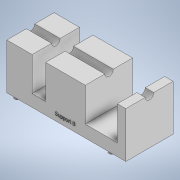
# Autodesk Inventor part: support_2
Saved by Autodesk Inventor 2021 (Build 250183000, 183)
## iProperties
Created: 2021-04-13
Part Number: support_2
Material: Generic
Document SubType Name: Modeling
Designer: Jawal
Density: 1 g/cm^3
Appearance: Default
Author: Jawal
Autodesk Inventor part; units mm, degrees
note: some values were not read from the file. Chosen so that the rebuilt part matches the saved one: direction of "Emboss1".
ref_plane "YZ Plane" through (0, 0, 0) normal (1, 0, 0) x (0, 1, 0)
ref_plane "XZ Plane" through (0, 0, 0) normal (0, 1, 0) x (-1, 0, 0)
ref_plane "XY Plane" through (0, 0, 0) normal (0, 0, 1) x (1, 0, 0)
sketch "Sketch7" plane through (0, 0, 0) normal (0, 1, 0) x (-1, 0, 0)
  line L0 (35, 14.012) -> (-35.5, 14.012)
  line L1 (-35.5, 14.012) -> (-35.5, -14.012)
  line L2 (-35.5, -14.012) -> (35, -14.012)
  line L3 (35, -14.012) -> (35, 14.012)
  point P0 (0, 0)
  dimension "d32" = 70.5
  dimension "d34" = 28.024
  dimension "d35" = 14.012
  constraints: 8 end point, 2 parallel, 1 horizontal, 1 perpendicular
  measures "d32" distance of L1.end L2.end
  measures "d34" distance of L2.end L0.start
  measures "d35" distance from line of L2 point (0, 0)
extrude "Extrusion3" add sketch "Sketch7" along normal blind 27.147
sketch "Sketch8" plane through (-35, 0, 14.012) normal (0, 0, 1) x (1, 0, 0)
  line L0 (70.5, 27.147) -> (0, 27.147) projected
  line L1 (15, 27.147) -> (23, 27.147)
  line L2 (23, 27.147) -> (23, 7.147)
  line L3 (23, 7.147) -> (15, 7.147)
  line L4 (15, 7.147) -> (15, 27.147)
  line L5 (0, 0) -> (0, 27.147) projected
  line L6 (46.5, 27.147) -> (65.5, 27.147)
  line L7 (65.5, 27.147) -> (65.5, 7.147)
  line L8 (65.5, 7.147) -> (46.5, 7.147)
  line L9 (46.5, 7.147) -> (46.5, 27.147)
  line L10 (70.5, 0) -> (70.5, 27.147) projected
  point P0 (35, 0)
  point P1 (23, 27.147)
  dimension "d39" = 20
  dimension "d40" = 15
  dimension "d41" = 8
  dimension "d42" = 46.5
  dimension "d44" = 5
  constraints: 16 end point, 4 parallel, 2 horizontal, 2 perpendicular, 2 point on line
  measures "d39" distance of L1.end L2.end
  measures "d40" distance between parallel lines of L5 L4
  measures "d41" distance of L2.end L3.end
  measures "d42" distance between parallel lines of L9 L5
  measures "d44" distance between parallel lines of L7 L10
extrude "Extrusion4" cut sketch "Sketch8" against normal through all
sketch "Sketch9" plane through (-35, 0, -14.012) normal (-1, 0, 0) x (0, 0, 1)
  line L0 (0, 27.147) -> (28.024, 27.147) projected
  arc A0 (11.512, 27.147) -> (16.512, 27.147) centre (14.012, 27.147) ccw
  point P0 (14.012, 0)
  dimension "d47" = 5
  constraints: 2 point on circle, 2 point on line, 1 centre point, 1 midpoint
  measures "d47" diameter of A0
extrude "Extrusion5" cut sketch "Sketch9" against normal through all
sketch "Sketch10" plane through (0, 0, 0) normal (0, -1, 0) x (1, 0, 0)
  circle A0 centre (-32.5, 10.512) radius 1.5
  line L0 (-35, -14.012) -> (-35, 14.012) projected
  circle A1 centre (23.5, 10.512) radius 1.5
  line L1 (35.5, 14.012) -> (35.5, -14.012) projected
  line L2 (-35, 14.012) -> (35.5, 14.012) projected
  point P0 (0, 0)
  dimension "d50" = 3
  dimension "d51" = 2.5
  dimension "d52" = 3
  dimension "d56" = 56
  dimension "d57" = 3.5
  dimension "d58" = 3.5
  constraints: 2 centre point
  measures "d50" diameter of A0
  measures "d51" distance from line of L0 A0.centre
  measures "d52" diameter of A1
  measures "d56" distance of A1.centre A0.centre
  measures "d57" distance from line of L2 A0.centre
  measures "d58" distance from line of L2 A1.centre
extrude "Extrusion6" add sketch "Sketch10" along normal blind 3
sketch "Sketch11" plane through (-35, 0, 14.012) normal (0, 0, 1) x (1, 0, 0)
  line L0 (28.6031, 5.0261) -> (50.5352, 5.0261) construction
  line L1 (50.5352, 5.0261) -> (50.5352, -0.6092) construction
  line L2 (50.5352, -0.6092) -> (28.6031, -0.6092) construction
  line L3 (28.6031, -0.6092) -> (28.6031, 5.0261) construction
  spline S0 degree 2 poles (29.3633, 2.9548) (29.1461, 2.9548) (28.8414, 3.0455) (28.7069, 3.1104) knots 0 0 0 1 2 2 2
  line L4 (28.7069, 3.1104) -> (28.7069, 3.4442)
  line L5 (28.7069, 3.4442) -> (28.7263, 3.4442)
  spline S1 degree 2 poles (28.7263, 3.4442) (28.8576, 3.3211) (29.1899, 3.1849) (29.3438, 3.1849) knots 0 0 0 1 2 2 2
  spline S2 degree 2 poles (29.3438, 3.1849) (29.5643, 3.1849) (29.7895, 3.3681) (29.7895, 3.5188) knots 0 0 0 1 2 2 2
  spline S3 degree 2 poles (29.7895, 3.5188) (29.7895, 3.6387) (29.6712, 3.7878) (29.5432, 3.8251) knots 0 0 0 1 2 2 2
  spline S4 degree 2 poles (29.5432, 3.8251) (29.4508, 3.8511) (29.2968, 3.8867) (29.1818, 3.9159) knots 0 0 0 1 2 2 2
  spline S5 degree 2 poles (29.1818, 3.9159) (29.078, 3.9434) (28.9143, 4.0261) (28.8511, 4.0925) knots 0 0 0 1 2 2 2
  spline S6 degree 2 poles (28.8511, 4.0925) (28.7895, 4.159) (28.7215, 4.3373) (28.7215, 4.454) knots 0 0 0 1 2 2 2
  spline S7 degree 2 poles (28.7215, 4.454) (28.7215, 4.6971) (29.1007, 5.0261) (29.3941, 5.0261) knots 0 0 0 1 2 2 2
  spline S8 degree 2 poles (29.3941, 5.0261) (29.5626, 5.0261) (29.8608, 4.9596) (29.9889, 4.8964) knots 0 0 0 1 2 2 2
  line L6 (29.9889, 4.8964) -> (29.9889, 4.5788)
  line L7 (29.9889, 4.5788) -> (29.9694, 4.5788)
  spline S9 degree 2 poles (29.9694, 4.5788) (29.8738, 4.6663) (29.5756, 4.796) (29.4119, 4.796) knots 0 0 0 1 2 2 2
  spline S10 degree 2 poles (29.4119, 4.796) (29.2271, 4.796) (28.9986, 4.6225) (28.9986, 4.4815) knots 0 0 0 1 2 2 2
  spline S11 degree 2 poles (28.9986, 4.4815) (28.9986, 4.3551) (29.1331, 4.2044) (29.2596, 4.1703) knots 0 0 0 1 2 2 2
  spline S12 degree 2 poles (29.2596, 4.1703) (29.3438, 4.1477) (29.5886, 4.0893) (29.6696, 4.065) knots 0 0 0 1 2 2 2
  spline S13 degree 2 poles (29.6696, 4.065) (29.8754, 4.0018) (30.0667, 3.7473) (30.0667, 3.5609) knots 0 0 0 1 2 2 2
  spline S14 degree 2 poles (30.0667, 3.5609) (30.0667, 3.4426) (29.9711, 3.2157) (29.8852, 3.1363) knots 0 0 0 1 2 2 2
  spline S15 degree 2 poles (29.8852, 3.1363) (29.7895, 3.0488) (29.5464, 2.9548) (29.3633, 2.9548) knots 0 0 0 1 2 2 2
  line L8 (31.4848, 2.9904) -> (31.232, 2.9904)
  line L9 (31.232, 2.9904) -> (31.232, 3.1558)
  spline S16 degree 2 poles (31.232, 3.1558) (31.1153, 3.0536) (30.9062, 2.9483) (30.7766, 2.9483) knots 0 0 0 1 2 2 2
  spline S17 degree 2 poles (30.7766, 2.9483) (30.6793, 2.9483) (30.5059, 3.0131) (30.4427, 3.0828) knots 0 0 0 1 2 2 2
  spline S18 degree 2 poles (30.4427, 3.0828) (30.3779, 3.1525) (30.3066, 3.3648) (30.3066, 3.5172) knots 0 0 0 1 2 2 2
  line L10 (30.3066, 3.5172) -> (30.3066, 4.4913)
  line L11 (30.3066, 4.4913) -> (30.5594, 4.4913)
  line L12 (30.5594, 4.4913) -> (30.5594, 3.6355)
  spline S19 degree 2 poles (30.5594, 3.6355) (30.5594, 3.5156) (30.5772, 3.3583) (30.608, 3.3) knots 0 0 0 1 2 2 2
  spline S20 degree 2 poles (30.608, 3.3) (30.6388, 3.2417) (30.7442, 3.1882) (30.843, 3.1882) knots 0 0 0 1 2 2 2
  spline S21 degree 2 poles (30.843, 3.1882) (30.9354, 3.1882) (31.1445, 3.2935) (31.232, 3.3697) knots 0 0 0 1 2 2 2
  line L13 (31.232, 3.3697) -> (31.232, 4.4913)
  line L14 (31.232, 4.4913) -> (31.4848, 4.4913)
  line L15 (31.4848, 4.4913) -> (31.4848, 2.9904)
  spline S22 degree 2 poles (33.1088, 3.7814) (33.1088, 3.4054) (32.7506, 2.9613) (32.4767, 2.9613) knots 0 0 0 1 2 2 2
  spline S23 degree 2 poles (32.4767, 2.9613) (32.3649, 2.9613) (32.1931, 3.0131) (32.104, 3.0666) knots 0 0 0 1 2 2 2
  line L16 (32.104, 3.0666) -> (32.104, 2.4378)
  line L17 (32.104, 2.4378) -> (31.8511, 2.4378)
  line L18 (31.8511, 2.4378) -> (31.8511, 4.4913)
  line L19 (31.8511, 4.4913) -> (32.104, 4.4913)
  line L20 (32.104, 4.4913) -> (32.104, 4.334)
  spline S24 degree 2 poles (32.104, 4.334) (32.198, 4.4199) (32.4281, 4.5334) (32.5626, 4.5334) knots 0 0 0 1 2 2 2
  spline S25 degree 2 poles (32.5626, 4.5334) (32.8203, 4.5334) (33.1088, 4.125) (33.1088, 3.7814) knots 0 0 0 1 2 2 2
  spline S26 degree 2 poles (32.8479, 3.7522) (32.8479, 4.0099) (32.6842, 4.2935) (32.501, 4.2935) knots 0 0 0 1 2 2 2
  spline S27 degree 2 poles (32.501, 4.2935) (32.3941, 4.2935) (32.1931, 4.1979) (32.104, 4.1233) knots 0 0 0 1 2 2 2
  line L21 (32.104, 4.1233) -> (32.104, 3.2708)
  spline S28 degree 2 poles (32.104, 3.2708) (32.2028, 3.2238) (32.3438, 3.1882) (32.4346, 3.1882) knots 0 0 0 1 2 2 2
  spline S29 degree 2 poles (32.4346, 3.1882) (32.6307, 3.1882) (32.8479, 3.4767) (32.8479, 3.7522) knots 0 0 0 1 2 2 2
  spline S30 degree 2 poles (34.6291, 3.7814) (34.6291, 3.4054) (34.2709, 2.9613) (33.997, 2.9613) knots 0 0 0 1 2 2 2
  spline S31 degree 2 poles (33.997, 2.9613) (33.8852, 2.9613) (33.7134, 3.0131) (33.6242, 3.0666) knots 0 0 0 1 2 2 2
  line L22 (33.6242, 3.0666) -> (33.6242, 2.4378)
  line L23 (33.6242, 2.4378) -> (33.3714, 2.4378)
  line L24 (33.3714, 2.4378) -> (33.3714, 4.4913)
  line L25 (33.3714, 4.4913) -> (33.6242, 4.4913)
  line L26 (33.6242, 4.4913) -> (33.6242, 4.334)
  spline S32 degree 2 poles (33.6242, 4.334) (33.7182, 4.4199) (33.9484, 4.5334) (34.0829, 4.5334) knots 0 0 0 1 2 2 2
  spline S33 degree 2 poles (34.0829, 4.5334) (34.3406, 4.5334) (34.6291, 4.125) (34.6291, 3.7814) knots 0 0 0 1 2 2 2
  spline S34 degree 2 poles (34.3681, 3.7522) (34.3681, 4.0099) (34.2044, 4.2935) (34.0213, 4.2935) knots 0 0 0 1 2 2 2
  spline S35 degree 2 poles (34.0213, 4.2935) (33.9143, 4.2935) (33.7134, 4.1979) (33.6242, 4.1233) knots 0 0 0 1 2 2 2
  line L27 (33.6242, 4.1233) -> (33.6242, 3.2708)
  spline S36 degree 2 poles (33.6242, 3.2708) (33.7231, 3.2238) (33.8641, 3.1882) (33.9549, 3.1882) knots 0 0 0 1 2 2 2
  spline S37 degree 2 poles (33.9549, 3.1882) (34.151, 3.1882) (34.3681, 3.4767) (34.3681, 3.7522) knots 0 0 0 1 2 2 2
  spline S38 degree 2 poles (36.125, 3.7408) (36.125, 3.3616) (35.7604, 2.9483) (35.4557, 2.9483) knots 0 0 0 1 2 2 2
  spline S39 degree 2 poles (35.4557, 2.9483) (35.1429, 2.9483) (34.7847, 3.3746) (34.7847, 3.7408) knots 0 0 0 1 2 2 2
  spline S40 degree 2 poles (34.7847, 3.7408) (34.7847, 4.1169) (35.1542, 4.5334) (35.4557, 4.5334) knots 0 0 0 1 2 2 2
  spline S41 degree 2 poles (35.4557, 4.5334) (35.7604, 4.5334) (36.125, 4.1185) (36.125, 3.7408) knots 0 0 0 1 2 2 2
  spline S42 degree 2 poles (35.8641, 3.7408) (35.8641, 4.0326) (35.6518, 4.3162) (35.4557, 4.3162) knots 0 0 0 1 2 2 2
  spline S43 degree 2 poles (35.4557, 4.3162) (35.2596, 4.3162) (35.0456, 4.0326) (35.0456, 3.7408) knots 0 0 0 1 2 2 2
  spline S44 degree 2 poles (35.0456, 3.7408) (35.0456, 3.4572) (35.2596, 3.1655) (35.4557, 3.1655) knots 0 0 0 1 2 2 2
  spline S45 degree 2 poles (35.4557, 3.1655) (35.6502, 3.1655) (35.8641, 3.4524) (35.8641, 3.7408) knots 0 0 0 1 2 2 2
  line L28 (37.1801, 4.2206) -> (37.1672, 4.2206)
  spline S46 degree 2 poles (37.1672, 4.2206) (37.138, 4.2287) (37.0748, 4.2319) (37.031, 4.2319) knots 0 0 0 1 2 2 2
  spline S47 degree 2 poles (37.031, 4.2319) (36.9289, 4.2319) (36.7279, 4.1428) (36.6372, 4.0553) knots 0 0 0 1 2 2 2
  line L29 (36.6372, 4.0553) -> (36.6372, 2.9904)
  line L30 (36.6372, 2.9904) -> (36.3843, 2.9904)
  line L31 (36.3843, 2.9904) -> (36.3843, 4.4913)
  line L32 (36.3843, 4.4913) -> (36.6372, 4.4913)
  line L33 (36.6372, 4.4913) -> (36.6372, 4.2676)
  spline S48 degree 2 poles (36.6372, 4.2676) (36.7749, 4.3908) (36.9808, 4.4913) (37.078, 4.4913) knots 0 0 0 1 2 2 2
  spline S49 degree 2 poles (37.078, 4.4913) (37.1169, 4.4913) (37.1558, 4.488) (37.1801, 4.4831) knots 0 0 0 1 2 2 2
  line L34 (37.1801, 4.4831) -> (37.1801, 4.2206)
  spline S50 degree 2 poles (37.8301, 2.9613) (37.6242, 2.9613) (37.3925, 3.1963) (37.3925, 3.4507) knots 0 0 0 1 2 2 2
  line L35 (37.3925, 3.4507) -> (37.3925, 4.2822)
  line L36 (37.3925, 4.2822) -> (37.2223, 4.2822)
  line L37 (37.2223, 4.2822) -> (37.2223, 4.4913)
  line L38 (37.2223, 4.4913) -> (37.3925, 4.4913)
  line L39 (37.3925, 4.4913) -> (37.3925, 4.9224)
  line L40 (37.3925, 4.9224) -> (37.6453, 4.9224)
  line L41 (37.6453, 4.9224) -> (37.6453, 4.4913)
  line L42 (37.6453, 4.4913) -> (38.1104, 4.4913)
  line L43 (38.1104, 4.4913) -> (38.1104, 4.2822)
  line L44 (38.1104, 4.2822) -> (37.6453, 4.2822)
  line L45 (37.6453, 4.2822) -> (37.6453, 3.5674)
  spline S51 degree 2 poles (37.6453, 3.5674) (37.6453, 3.454) (37.6534, 3.3292) (37.6809, 3.2757) knots 0 0 0 1 2 2 2
  spline S52 degree 2 poles (37.6809, 3.2757) (37.7036, 3.2287) (37.8057, 3.1817) (37.8933, 3.1817) knots 0 0 0 1 2 2 2
  spline S53 degree 2 poles (37.8933, 3.1817) (37.9549, 3.1817) (38.0699, 3.219) (38.0959, 3.2303) knots 0 0 0 1 2 2 2
  line L46 (38.0959, 3.2303) -> (38.1104, 3.2303)
  line L47 (38.1104, 3.2303) -> (38.1104, 3.0034)
  spline S54 degree 2 poles (38.1104, 3.0034) (38.0391, 2.984) (37.8933, 2.9613) (37.8301, 2.9613) knots 0 0 0 1 2 2 2
  spline S55 degree 2 poles (40.5318, 3.6047) (40.5318, 3.4556) (40.4184, 3.2271) (40.3244, 3.1525) knots 0 0 0 1 2 2 2
  spline S56 degree 2 poles (40.3244, 3.1525) (40.2109, 3.065) (39.9532, 2.9904) (39.749, 2.9904) knots 0 0 0 1 2 2 2
  line L48 (39.749, 2.9904) -> (39.1753, 2.9904)
  line L49 (39.1753, 2.9904) -> (39.1753, 4.9904)
  line L50 (39.1753, 4.9904) -> (39.7053, 4.9904)
  spline S57 degree 2 poles (39.7053, 4.9904) (39.9192, 4.9904) (40.1331, 4.9629) (40.2304, 4.9094) knots 0 0 0 1 2 2 2
  spline S58 degree 2 poles (40.2304, 4.9094) (40.339, 4.8527) (40.4378, 4.6663) (40.4378, 4.5399) knots 0 0 0 1 2 2 2
  spline S59 degree 2 poles (40.4378, 4.5399) (40.4378, 4.3989) (40.2887, 4.1752) (40.1574, 4.112) knots 0 0 0 1 2 2 2
  line L51 (40.1574, 4.112) -> (40.1574, 4.1023)
  spline S60 degree 2 poles (40.1574, 4.1023) (40.3357, 4.0536) (40.5318, 3.796) (40.5318, 3.6047) knots 0 0 0 1 2 2 2
  spline S61 degree 2 poles (40.2547, 3.5934) (40.2547, 3.7068) (40.1899, 3.8527) (40.0926, 3.9045) knots 0 0 0 1 2 2 2
  spline S62 degree 2 poles (40.0926, 3.9045) (40.0294, 3.937) (39.8803, 3.9564) (39.7425, 3.9564) knots 0 0 0 1 2 2 2
  line L52 (39.7425, 3.9564) -> (39.4411, 3.9564)
  line L53 (39.4411, 3.9564) -> (39.4411, 3.2173)
  line L54 (39.4411, 3.2173) -> (39.6566, 3.2173)
  spline S63 degree 2 poles (39.6566, 3.2173) (39.8317, 3.2173) (40.0326, 3.2498) (40.1104, 3.3016) knots 0 0 0 1 2 2 2
  spline S64 degree 2 poles (40.1104, 3.3016) (40.185, 3.3551) (40.2547, 3.488) (40.2547, 3.5934) knots 0 0 0 1 2 2 2
  spline S65 degree 2 poles (40.1607, 4.5026) (40.1607, 4.5739) (40.1121, 4.6809) (40.0586, 4.7117) knots 0 0 0 1 2 2 2
  spline S66 degree 2 poles (40.0586, 4.7117) (39.9937, 4.7473) (39.8365, 4.7635) (39.6955, 4.7635) knots 0 0 0 1 2 2 2
  line L55 (39.6955, 4.7635) -> (39.4411, 4.7635)
  line L56 (39.4411, 4.7635) -> (39.4411, 4.1784)
  line L57 (39.4411, 4.1784) -> (39.7425, 4.1784)
  spline S67 degree 2 poles (39.7425, 4.1784) (39.8673, 4.1784) (39.9856, 4.2044) (40.0489, 4.2449) knots 0 0 0 1 2 2 2
  spline S68 degree 2 poles (40.0489, 4.2449) (40.1104, 4.2838) (40.1607, 4.4086) (40.1607, 4.5026) knots 0 0 0 1 2 2 2
  point P0 (35, 0)
  constraints: 2 other
emboss "Emboss1" sketch "Sketch11" operation cut depth 1 direction (0, 0, -1)
equation "\"d35\" = 0.5 * d34"
body "Solid2"
